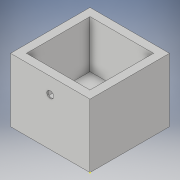
# Autodesk Inventor part: lampbottom
Saved by Autodesk Inventor 2019 (Build 230136000, 136)
## iProperties
Created: 2019-08-13
Part Number: lampbottom
Material: Generic
Document SubType Name: Modeling
Designer: Riley
Density: 1 g/cm^3
Appearance: Default
Author: Riley
Autodesk Inventor part; units mm, degrees
ref_plane "YZ Plane" through (0, 0, 0) normal (1, 0, 0) x (0, 1, 0)
ref_plane "XZ Plane" through (0, 0, 0) normal (0, 1, 0) x (-1, 0, 0)
ref_plane "XY Plane" through (0, 0, 0) normal (0, 0, 1) x (1, 0, 0)
sketch "Sketch1" plane through (0, 0, 0) normal (0, 1, 0) x (-1, 0, 0)
  line L0 (0, 0) -> (127, 0)
  line L1 (127, 0) -> (127, -127)
  line L2 (127, -127) -> (0, -127)
  line L3 (0, -127) -> (0, 0)
  dimension "d0" = 127
  dimension "d1" = 127
  constraints: 8 end point, 2 parallel, 1 horizontal, 1 perpendicular
  measures "d0" distance of L1.end L2.end
  measures "d1" distance of L0.end L1.end
extrude "Extrusion1" add sketch "Sketch1" along normal blind 101.6
sketch "Sketch2" plane through (0, 101.6, 0) normal (0, 1, 0) x (1, 0, 0)
  line L0 (-114.3, 114.3) -> (-12.7, 114.3)
  line L1 (-12.7, 114.3) -> (-12.7, 12.7)
  line L2 (-12.7, 12.7) -> (-114.3, 12.7)
  line L3 (-114.3, 12.7) -> (-114.3, 114.3)
  line L4 (-127, 127) -> (-127, 0) projected
  line L5 (0, 127) -> (-127, 127) projected
  point P0 (0, 0)
  dimension "d4" = 101.6
  dimension "d5" = 101.6
  dimension "d6" = 12.7
  dimension "d7" = 12.7
  constraints: 8 end point, 2 parallel, 1 horizontal, 1 perpendicular
  measures "d4" distance between parallel lines of L2 L0
  measures "d5" distance between parallel lines of L1 L3
  measures "d6" distance between parallel lines of L4 L3
  measures "d7" distance between parallel lines of L5 L0
extrude "Extrusion2" cut sketch "Sketch2" against normal blind 76.2
sketch "Sketch3" plane through (-127, 0, 0) normal (0, 0, 1) x (1, 0, 0)
  point P0 (127, 0)
sketch "Sketch4" plane through (-127, 0, 0) normal (0, 0, 1) x (1, 0, 0)
  circle A0 centre (63.5, 76.2) radius 5.4991
  line L0 (127, 0) -> (0, 0) projected
  line L1 (127, 0) -> (127, 101.6) projected
  dimension "d10" = 10.9982
  dimension "d11" = 76.2
  dimension "d12" = 63.5
  constraints: 1 centre point
  measures "d10" diameter of A0
  measures "d11" distance from line of L0 A0.centre
  measures "d12" distance from line of L1 A0.centre
extrude "Extrusion3" cut sketch "Sketch4" against normal blind 76.2
sketch "Sketch5" plane through (-12.7, 101.6, -12.7) normal (0, 0, -1) x (-1, 0, 0)
  circle A0 centre (50.8, -25.4) radius 17.78
  line L0 (0, -76.2) -> (101.6, -76.2) projected
  line L1 (0, 0) -> (0, -76.2) projected
  point P0 (-12.7, -101.6)
  dimension "d15" = 35.56
  dimension "d16" = 50.8
  dimension "d17" = 50.8
  constraints: 1 centre point
  measures "d15" diameter of A0
  measures "d16" distance from line of L0 A0.centre
  measures "d17" distance from line of L1 A0.centre
extrude "Extrusion4" cut sketch "Sketch5" against normal blind 10.795
chamfer "Chamfer2" distance 10.795 angle 30 1 edges at (-45.72, 76.2, -12.7) measured on face at (-45.72, 76.2, -12.2)
sketch "Sketch6" plane through (0, 0, 0) normal (0, -1, 0) x (1, 0, 0)
  line L0 (-57.2968, -57.2968) -> (-69.7032, -57.2968)
  line L1 (-69.7032, -57.2968) -> (-69.7032, -69.7032)
  line L2 (-69.7032, -69.7032) -> (-57.2968, -69.7032)
  line L3 (-57.2968, -69.7032) -> (-57.2968, -57.2968)
  line L4 (-127, -127) -> (0, -127) projected
  line L5 (0, -127) -> (0, 0) projected
  line L6 (0, 0) -> (-127, 0) projected
  line L7 (-127, 0) -> (-127, -127) projected
  dimension "d26" = 12.4064
  dimension "d27" = 12.4064
  dimension "d28" = 57.2968
  dimension "d29" = 57.2968
  dimension "d30" = 57.2968
  dimension "d31" = 57.2968
  constraints: 8 end point, 2 parallel, 1 horizontal, 1 perpendicular
  measures "d26" distance of L2.end L1.end
  measures "d27" distance of L1.end L0.end
  measures "d28" distance between parallel lines of L4 L2
  measures "d29" distance between parallel lines of L5 L3
  measures "d30" distance between parallel lines of L6 L0
  measures "d31" distance between parallel lines of L7 L1
extrude "Extrusion5" cut sketch "Sketch6" against normal blind 25.4 contours L3 L2 L1 L0
equation "\"d6\" = -0.5 * d4 + 0.5 * d1"
equation "\"d7\" = -0.5 * d5 + 0.5 * d0"
equation "\"d12\" = 0.5 * d0"
equation "\"d28\" = -0.5 * d27 + 0.5 * d1"
equation "\"d29\" = -0.5 * d26 + 0.5 * d0"
body "Solid1"
